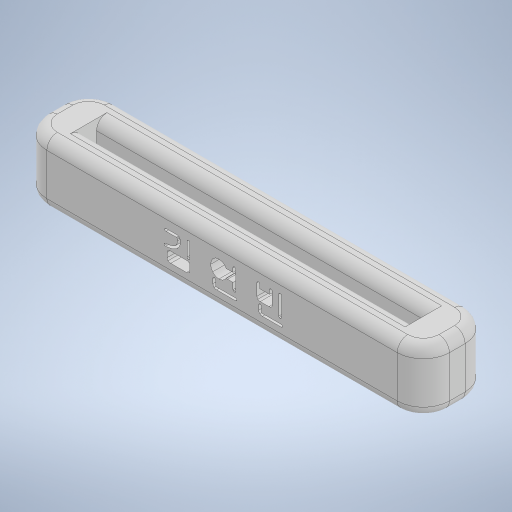
# Autodesk Inventor part: part2
Saved by Autodesk Inventor 2024 (Build 280153000, 153)
## iProperties
Created: 2023-11-09
Part Number: part2
Material: 일반
Document SubType Name: Modeling
Designer: SSAFY
Density: 1 g/cm^3
Appearance: 기본값
Author: SSAFY
Autodesk Inventor part; units mm, degrees
ref_plane "YZ Plane" through (0, 0, 0) normal (1, 0, 0) x (0, 1, 0)
ref_plane "XZ Plane" through (0, 0, 0) normal (0, 1, 0) x (-1, 0, 0)
ref_plane "XY Plane" through (0, 0, 0) normal (0, 0, 1) x (1, 0, 0)
sketch "스케치1" plane through (0, 0, 0) normal (0, 0, 1) x (1, 0, 0)
  point P0 (0, 0)
sketch "스케치2" plane through (0, 0, 0) normal (0, 1, 0) x (-1, 0, 0)
  line L0 (-38.5, 6.5) -> (38.5, 6.5)
  line L1 (38.5, 6.5) -> (38.5, -6.5)
  line L2 (38.5, -6.5) -> (-38.5, -6.5)
  line L3 (-38.5, -6.5) -> (-38.5, 6.5)
  line L4 (-38.5, 6.5) -> (38.5, -6.5) construction
  line L5 (38.5, 6.5) -> (-38.5, -6.5) construction
  line L6 (-32, 1.5) -> (32, 1.5)
  line L7 (32, 1.5) -> (32, -1.5)
  line L8 (32, -1.5) -> (-32, -1.5)
  line L9 (-32, -1.5) -> (-32, 1.5)
  line L10 (-32, 1.5) -> (32, -1.5) construction
  line L11 (32, 1.5) -> (-32, -1.5) construction
  point P0 (0, 0)
  dimension "d0" = 77
  dimension "d1" = 13
  dimension "d2" = 64
  dimension "d3" = 3
  constraints: 24 end point, 4 midpoint, 4 parallel, 2 horizontal, 2 perpendicular
  measures "d0" distance of L1.end L2.end
  measures "d1" distance of L2.end L0.start
  measures "d2" distance of L7.end L8.end
  measures "d3" distance of L8.end L6.start
extrude "돌출1" add sketch "스케치2" along normal mid plane 12
fillet "모깎기1" radius 5 4 edges at (38.5, 0, 6.5) (38.5, 0, -6.5) (-38.5, 0, 6.5) (-38.5, 0, -6.5)
fillet "모깎기2" radius 2 20 edges at (0, 6, 1.5) (0, -6, 1.5) (0, -6, -1.5) (0, 6, -1.5) (-37.0355, 6, -5.0355) (-38.5, 6, 0) (-37.0355, 6, 5.0355) (0, 6, 6.5) (37.0355, 6, 5.0355) (38.5, 6, 0) (37.0355, 6, -5.0355) (0, 6, -6.5) (37.0355, -6, -5.0355) (38.5, -6, 0) (37.0355, -6, 5.0355) (0, -6, 6.5) (-37.0355, -6, 5.0355) (-38.5, -6, 0) (-37.0355, -6, -5.0355) (0, -6, -6.5)
sketch "스케치3" plane through (-33.5, -4, 6.5) normal (0, 0, 1) x (1, 0, 0)
  line L0 (17.2421, 7.3141) -> (50.5083, 7.3141) construction
  line L1 (50.5083, 7.3141) -> (50.5083, 0.4358) construction
  line L2 (50.5083, 0.4358) -> (17.2421, 0.4358) construction
  line L3 (17.2421, 0.4358) -> (17.2421, 7.3141) construction
  line L4 (26.7014, 3.1578) -> (23.6098, 3.1578)
  spline S0 degree 2 poles (23.6098, 3.1578) (23.3343, 3.1578) (23.1722, 2.9997) knots 0 0 0 1 1 1
  spline S1 degree 2 poles (23.1722, 2.9997) (23.0061, 2.8417) (23.0061, 2.6067) knots 0 0 0 1 1 1
  line L5 (23.0061, 2.6067) -> (23.0061, 1.7396)
  spline S2 degree 2 poles (23.0061, 1.7396) (23.0061, 1.4479) (23.1641, 1.2939) knots 0 0 0 1 1 1
  spline S3 degree 2 poles (23.1641, 1.2939) (23.3343, 1.1318) (23.6949, 1.1318) knots 0 0 0 1 1 1
  line L6 (23.6949, 1.1318) -> (26.7297, 1.1318)
  spline S4 degree 2 poles (26.7297, 1.1318) (27.0174, 1.1318) (27.2119, 1.3749) knots 0 0 0 1 1 1
  spline S5 degree 2 poles (27.2119, 1.3749) (27.3699, 1.4236) (27.3699, 1.7072) knots 0 0 0 1 1 1
  line L7 (27.3699, 1.7072) -> (27.3699, 2.631)
  spline S6 degree 2 poles (27.3699, 2.631) (27.3699, 2.8701) (27.2119, 2.9997) knots 0 0 0 1 1 1
  spline S7 degree 2 poles (27.2119, 2.9997) (27.0012, 3.1578) (26.7014, 3.1578) knots 0 0 0 1 1 1
  line L8 (26.8351, 2.5338) -> (26.8351, 1.7477)
  spline S8 degree 2 poles (26.8351, 1.7477) (26.8351, 1.6667) (26.8027, 1.6424) knots 0 0 0 1 1 1
  spline S9 degree 2 poles (26.8027, 1.6424) (26.7419, 1.6018) (26.6163, 1.6018) knots 0 0 0 1 1 1
  line L9 (26.6163, 1.6018) -> (23.7678, 1.6018)
  spline S10 degree 2 poles (23.7678, 1.6018) (23.6219, 1.6018) (23.5733, 1.6424) knots 0 0 0 1 1 1
  spline S11 degree 2 poles (23.5733, 1.6424) (23.5409, 1.6707) (23.5409, 1.7761) knots 0 0 0 1 1 1
  line L10 (23.5409, 1.7761) -> (23.5409, 2.5176)
  spline S12 degree 2 poles (23.5409, 2.5176) (23.5409, 2.6148) (23.5814, 2.6553) knots 0 0 0 1 1 1
  spline S13 degree 2 poles (23.5814, 2.6553) (23.6179, 2.6877) (23.7475, 2.6877) knots 0 0 0 1 1 1
  line L11 (23.7475, 2.6877) -> (26.6082, 2.6877)
  spline S14 degree 2 poles (26.6082, 2.6877) (26.7419, 2.6877) (26.8027, 2.6472) knots 0 0 0 1 1 1
  spline S15 degree 2 poles (26.8027, 2.6472) (26.8351, 2.6229) (26.8351, 2.5338) knots 0 0 0 1 1 1
  line L12 (24.8051, 6.46) -> (22.7913, 6.46)
  spline S16 degree 2 poles (22.7913, 6.46) (22.536, 6.46) (22.5441, 6.2291) knots 0 0 0 1 1 1
  spline S17 degree 2 poles (22.5441, 6.2291) (22.5441, 5.99) (22.7954, 5.99) knots 0 0 0 1 1 1
  line L13 (22.7954, 5.99) -> (24.7646, 5.99)
  spline S18 degree 2 poles (24.7646, 5.99) (24.878, 5.99) (24.9307, 5.9454) knots 0 0 0 1 1 1
  spline S19 degree 2 poles (24.9307, 5.9454) (24.9996, 5.8928) (24.9996, 5.7874) knots 0 0 0 1 1 1
  line L14 (24.9996, 5.7874) -> (24.9996, 5.4997)
  spline S20 degree 2 poles (24.9996, 5.4997) (24.9996, 4.7907) (24.489, 4.4098) knots 0 0 0 1 1 1
  spline S21 degree 2 poles (24.489, 4.4098) (23.8286, 4.0046) (22.7305, 3.96) knots 0 0 0 1 1 1
  spline S22 degree 2 poles (22.7305, 3.96) (22.5766, 3.96) (22.4996, 3.883) knots 0 0 0 1 1 1
  spline S23 degree 2 poles (22.4996, 3.883) (22.4347, 3.8142) (22.4347, 3.7169) knots 0 0 0 1 1 1
  spline S24 degree 2 poles (22.4347, 3.7169) (22.4347, 3.6156) (22.5198, 3.5508) knots 0 0 0 1 1 1
  spline S25 degree 2 poles (22.5198, 3.5508) (22.5968, 3.49) (22.7224, 3.49) knots 0 0 0 1 1 1
  spline S26 degree 2 poles (22.7224, 3.49) (24.0393, 3.5508) (24.7727, 4.0816) knots 0 0 0 1 1 1
  spline S27 degree 2 poles (24.7727, 4.0816) (25.5142, 4.6164) (25.5142, 5.4957) knots 0 0 0 1 1 1
  line L15 (25.5142, 5.4957) -> (25.5142, 5.8441)
  spline S28 degree 2 poles (25.5142, 5.8441) (25.5142, 6.1197) (25.2994, 6.298) knots 0 0 0 1 1 1
  spline S29 degree 2 poles (25.2994, 6.298) (25.109, 6.46) (24.8051, 6.46) knots 0 0 0 1 1 1
  line L16 (27.3699, 3.7493) -> (27.3699, 6.3749)
  spline S30 degree 2 poles (27.3699, 6.3749) (27.3699, 6.4924) (27.2767, 6.5573) knots 0 0 0 1 1 1
  spline S31 degree 2 poles (27.2767, 6.5573) (27.2078, 6.6181) (27.1025, 6.6181) knots 0 0 0 1 1 1
  spline S32 degree 2 poles (27.1025, 6.6181) (26.989, 6.6181) (26.9161, 6.5573) knots 0 0 0 1 1 1
  spline S33 degree 2 poles (26.9161, 6.5573) (26.8351, 6.4803) (26.8351, 6.3709) knots 0 0 0 1 1 1
  line L17 (26.8351, 6.3709) -> (26.8351, 3.7493)
  spline S34 degree 2 poles (26.8351, 3.7493) (26.8351, 3.6278) (26.9121, 3.5508) knots 0 0 0 1 1 1
  spline S35 degree 2 poles (26.9121, 3.5508) (26.985, 3.4779) (27.1025, 3.4779) knots 0 0 0 1 1 1
  spline S36 degree 2 poles (27.1025, 3.4779) (27.2119, 3.4779) (27.2929, 3.5589) knots 0 0 0 1 1 1
  spline S37 degree 2 poles (27.2929, 3.5589) (27.3699, 3.6278) (27.3699, 3.7493) knots 0 0 0 1 1 1
  spline S38 degree 2 poles (32.921, 6.4479) (32.1714, 6.4479) (31.7297, 5.9292) knots 0 0 0 1 1 1
  spline S39 degree 2 poles (31.7297, 5.9292) (31.3367, 5.4714) (31.3367, 4.8028) knots 0 0 0 1 1 1
  spline S40 degree 2 poles (31.3367, 4.8028) (31.3367, 4.1383) (31.7135, 3.7412) knots 0 0 0 1 1 1
  spline S41 degree 2 poles (31.7135, 3.7412) (32.1714, 3.1537) (32.921, 3.1537) knots 0 0 0 1 1 1
  spline S42 degree 2 poles (32.921, 3.1537) (33.6584, 3.1537) (34.092, 3.6723) knots 0 0 0 1 1 1
  spline S43 degree 2 poles (34.092, 3.6723) (34.485, 4.1343) (34.485, 4.8028) knots 0 0 0 1 1 1
  spline S44 degree 2 poles (34.485, 4.8028) (34.485, 5.4714) (34.092, 5.9292) knots 0 0 0 1 1 1
  spline S45 degree 2 poles (34.092, 5.9292) (33.6584, 6.4479) (32.921, 6.4479) knots 0 0 0 1 1 1
  spline S46 degree 2 poles (32.921, 5.9779) (33.4193, 5.9779) (33.6989, 5.6213) knots 0 0 0 1 1 1
  spline S47 degree 2 poles (33.6989, 5.6213) (33.9664, 5.289) (33.9664, 4.8028) knots 0 0 0 1 1 1
  spline S48 degree 2 poles (33.9664, 4.8028) (33.9664, 4.3125) (33.6949, 3.9762) knots 0 0 0 1 1 1
  spline S49 degree 2 poles (33.6949, 3.9762) (33.4193, 3.6237) (32.921, 3.6237) knots 0 0 0 1 1 1
  spline S50 degree 2 poles (32.921, 3.6237) (32.4104, 3.6237) (32.1268, 3.9884) knots 0 0 0 1 1 1
  spline S51 degree 2 poles (32.1268, 3.9884) (31.8715, 4.3085) (31.8715, 4.8028) knots 0 0 0 1 1 1
  spline S52 degree 2 poles (31.8715, 4.8028) (31.8715, 5.2931) (32.1268, 5.6172) knots 0 0 0 1 1 1
  spline S53 degree 2 poles (32.1268, 5.6172) (32.4145, 5.9779) (32.921, 5.9779) knots 0 0 0 1 1 1
  line L18 (36.13, 2.7404) -> (36.13, 6.3749)
  spline S54 degree 2 poles (36.13, 6.3749) (36.13, 6.4924) (36.0409, 6.5532) knots 0 0 0 1 1 1
  spline S55 degree 2 poles (36.0409, 6.5532) (35.968, 6.6181) (35.8626, 6.6181) knots 0 0 0 1 1 1
  spline S56 degree 2 poles (35.8626, 6.6181) (35.7492, 6.6181) (35.6762, 6.5573) knots 0 0 0 1 1 1
  spline S57 degree 2 poles (35.6762, 6.5573) (35.5952, 6.4843) (35.5952, 6.3709) knots 0 0 0 1 1 1
  line L19 (35.5952, 6.3709) -> (35.5952, 5.5929)
  line L20 (35.5952, 5.5929) -> (34.5417, 5.5929)
  spline S58 degree 2 poles (34.5417, 5.5929) (34.4121, 5.5929) (34.3391, 5.5281) knots 0 0 0 1 1 1
  spline S59 degree 2 poles (34.3391, 5.5281) (34.2743, 5.4552) (34.2743, 5.3539) knots 0 0 0 1 1 1
  spline S60 degree 2 poles (34.2743, 5.3539) (34.2824, 5.2647) (34.3513, 5.1958) knots 0 0 0 1 1 1
  spline S61 degree 2 poles (34.3513, 5.1958) (34.4445, 5.1229) (34.5741, 5.1229) knots 0 0 0 1 1 1
  line L21 (34.5741, 5.1229) -> (35.5952, 5.1229)
  line L22 (35.5952, 5.1229) -> (35.5952, 4.3936)
  line L23 (35.5952, 4.3936) -> (34.5539, 4.3936)
  spline S62 degree 2 poles (34.5539, 4.3936) (34.4323, 4.3936) (34.3472, 4.3287) knots 0 0 0 1 1 1
  spline S63 degree 2 poles (34.3472, 4.3287) (34.2824, 4.2639) (34.2824, 4.1667) knots 0 0 0 1 1 1
  spline S64 degree 2 poles (34.2824, 4.1667) (34.2824, 4.0654) (34.3594, 4.0005) knots 0 0 0 1 1 1
  spline S65 degree 2 poles (34.3594, 4.0005) (34.4364, 3.9317) (34.562, 3.9317) knots 0 0 0 1 1 1
  line L24 (34.562, 3.9317) -> (35.5952, 3.9317)
  line L25 (35.5952, 3.9317) -> (35.5952, 2.7404)
  spline S66 degree 2 poles (35.5952, 2.7404) (35.5952, 2.6108) (35.6722, 2.5338) knots 0 0 0 1 1 1
  spline S67 degree 2 poles (35.6722, 2.5338) (35.7451, 2.4608) (35.8626, 2.4608) knots 0 0 0 1 1 1
  spline S68 degree 2 poles (35.8626, 2.4608) (35.972, 2.4608) (36.0531, 2.5419) knots 0 0 0 1 1 1
  spline S69 degree 2 poles (36.0531, 2.5419) (36.13, 2.6108) (36.13, 2.7404) knots 0 0 0 1 1 1
  spline S70 degree 2 poles (32.2929, 2.6634) (32.2929, 2.7971) (32.2159, 2.866) knots 0 0 0 1 1 1
  spline S71 degree 2 poles (32.2159, 2.866) (32.1349, 2.9471) (32.0255, 2.9471) knots 0 0 0 1 1 1
  spline S72 degree 2 poles (32.0255, 2.9471) (31.908, 2.9471) (31.8351, 2.8741) knots 0 0 0 1 1 1
  spline S73 degree 2 poles (31.8351, 2.8741) (31.7581, 2.7971) (31.7581, 2.6634) knots 0 0 0 1 1 1
  line L26 (31.7581, 2.6634) -> (31.7581, 1.7882)
  spline S74 degree 2 poles (31.7581, 1.7882) (31.7581, 1.4641) (31.9728, 1.2858) knots 0 0 0 1 1 1
  spline S75 degree 2 poles (31.9728, 1.2858) (32.1552, 1.1318) (32.4793, 1.1318) knots 0 0 0 1 1 1
  line L27 (32.4793, 1.1318) -> (36.0936, 1.1318)
  spline S76 degree 2 poles (36.0936, 1.1318) (36.3286, 1.1318) (36.3286, 1.3709) knots 0 0 0 1 1 1
  spline S77 degree 2 poles (36.3286, 1.3709) (36.3286, 1.6018) (36.0936, 1.6018) knots 0 0 0 1 1 1
  line L28 (36.0936, 1.6018) -> (32.5482, 1.6018)
  spline S78 degree 2 poles (32.5482, 1.6018) (32.3821, 1.6018) (32.3456, 1.6343) knots 0 0 0 1 1 1
  spline S79 degree 2 poles (32.3456, 1.6343) (32.2929, 1.6869) (32.2929, 1.8409) knots 0 0 0 1 1 1
  line L29 (32.2929, 1.8409) -> (32.2929, 2.6634)
  line L30 (42.5887, 6.2048) -> (42.5887, 5.4471)
  line L31 (42.5887, 5.4471) -> (40.7046, 5.4471)
  line L32 (40.7046, 5.4471) -> (40.7046, 6.1723)
  spline S80 degree 2 poles (40.7046, 6.1723) (40.7046, 6.3061) (40.6276, 6.3749) knots 0 0 0 1 1 1
  spline S81 degree 2 poles (40.6276, 6.3749) (40.5466, 6.456) (40.4372, 6.456) knots 0 0 0 1 1 1
  spline S82 degree 2 poles (40.4372, 6.456) (40.3278, 6.456) (40.2629, 6.383) knots 0 0 0 1 1 1
  spline S83 degree 2 poles (40.2629, 6.383) (40.1779, 6.298) (40.1779, 6.1683) knots 0 0 0 1 1 1
  line L33 (40.1779, 6.1683) -> (40.1779, 3.9276)
  spline S84 degree 2 poles (40.1779, 3.9276) (40.1779, 3.6521) (40.344, 3.5062) knots 0 0 0 1 1 1
  spline S85 degree 2 poles (40.344, 3.5062) (40.5304, 3.3522) (40.8018, 3.3522) knots 0 0 0 1 1 1
  line L34 (40.8018, 3.3522) -> (42.455, 3.3522)
  spline S86 degree 2 poles (42.455, 3.3522) (42.7386, 3.3522) (42.9129, 3.5103) knots 0 0 0 1 1 1
  spline S87 degree 2 poles (42.9129, 3.5103) (43.1033, 3.6723) (43.1033, 3.9276) knots 0 0 0 1 1 1
  line L35 (43.1033, 3.9276) -> (43.1033, 6.2007)
  spline S88 degree 2 poles (43.1033, 6.2007) (43.1033, 6.456) (42.844, 6.456) knots 0 0 0 1 1 1
  spline S89 degree 2 poles (42.844, 6.456) (42.5887, 6.456) (42.5887, 6.2048) knots 0 0 0 1 1 1
  spline S90 degree 2 poles (41.0531, 2.6634) (41.0531, 2.7971) (40.9761, 2.866) knots 0 0 0 1 1 1
  spline S91 degree 2 poles (40.9761, 2.866) (40.895, 2.9471) (40.7856, 2.9471) knots 0 0 0 1 1 1
  spline S92 degree 2 poles (40.7856, 2.9471) (40.6681, 2.9471) (40.5952, 2.8741) knots 0 0 0 1 1 1
  spline S93 degree 2 poles (40.5952, 2.8741) (40.5182, 2.7971) (40.5182, 2.6634) knots 0 0 0 1 1 1
  line L36 (40.5182, 2.6634) -> (40.5182, 1.7882)
  spline S94 degree 2 poles (40.5182, 1.7882) (40.5182, 1.4641) (40.733, 1.2858) knots 0 0 0 1 1 1
  spline S95 degree 2 poles (40.733, 1.2858) (40.9153, 1.1318) (41.2394, 1.1318) knots 0 0 0 1 1 1
  line L37 (41.2394, 1.1318) -> (44.8537, 1.1318)
  spline S96 degree 2 poles (44.8537, 1.1318) (45.0887, 1.1318) (45.0887, 1.3709) knots 0 0 0 1 1 1
  spline S97 degree 2 poles (45.0887, 1.3709) (45.0887, 1.6018) (44.8537, 1.6018) knots 0 0 0 1 1 1
  line L38 (44.8537, 1.6018) -> (41.3083, 1.6018)
  spline S98 degree 2 poles (41.3083, 1.6018) (41.1422, 1.6018) (41.1057, 1.6343) knots 0 0 0 1 1 1
  spline S99 degree 2 poles (41.1057, 1.6343) (41.0531, 1.6869) (41.0531, 1.8409) knots 0 0 0 1 1 1
  line L39 (41.0531, 1.8409) -> (41.0531, 2.6634)
  line L40 (44.8902, 2.7404) -> (44.8902, 6.3749)
  spline S100 degree 2 poles (44.8902, 6.3749) (44.8902, 6.4924) (44.801, 6.5532) knots 0 0 0 1 1 1
  spline S101 degree 2 poles (44.801, 6.5532) (44.7281, 6.6181) (44.6228, 6.6181) knots 0 0 0 1 1 1
  spline S102 degree 2 poles (44.6228, 6.6181) (44.5093, 6.6181) (44.4364, 6.5573) knots 0 0 0 1 1 1
  spline S103 degree 2 poles (44.4364, 6.5573) (44.3553, 6.4803) (44.3553, 6.3709) knots 0 0 0 1 1 1
  line L41 (44.3553, 6.3709) -> (44.3553, 2.7404)
  spline S104 degree 2 poles (44.3553, 2.7404) (44.3553, 2.6108) (44.4323, 2.5338) knots 0 0 0 1 1 1
  spline S105 degree 2 poles (44.4323, 2.5338) (44.5052, 2.4608) (44.6228, 2.4608) knots 0 0 0 1 1 1
  spline S106 degree 2 poles (44.6228, 2.4608) (44.7322, 2.4608) (44.8132, 2.5419) knots 0 0 0 1 1 1
  spline S107 degree 2 poles (44.8132, 2.5419) (44.8902, 2.6108) (44.8902, 2.7404) knots 0 0 0 1 1 1
  line L42 (42.5887, 4.977) -> (42.5887, 4.0087)
  spline S108 degree 2 poles (42.5887, 4.0087) (42.5887, 3.9074) (42.5279, 3.8668) knots 0 0 0 1 1 1
  spline S109 degree 2 poles (42.5279, 3.8668) (42.4753, 3.8223) (42.3416, 3.8223) knots 0 0 0 1 1 1
  line L43 (42.3416, 3.8223) -> (40.9072, 3.8223)
  spline S110 degree 2 poles (40.9072, 3.8223) (40.7816, 3.8223) (40.7492, 3.8547) knots 0 0 0 1 1 1
  spline S111 degree 2 poles (40.7492, 3.8547) (40.7046, 3.8911) (40.7046, 4.0087) knots 0 0 0 1 1 1
  line L44 (40.7046, 4.0087) -> (40.7046, 4.977)
  line L45 (40.7046, 4.977) -> (42.5887, 4.977)
  point P0 (33.5, 4)
  constraints: 2 other
emboss "엠보싱1" sketch "스케치3" operation cut depth 5 direction (0, 0, -1) contours S7 S6 L7 S5 S4 L6 S3 S2 L5 S1 S0 L4 | S29 S28 L15 S27 S26 S25 S24 S23 S22 S21 S20 L14 S19 S18 L13 S17 S16 L12 | S37 S36 S35 S34 L17 S33 S32 S31 S30 L16 | S45 S44 S58 S59 S60 S61 S43 S62 S63 S64 S42 S41 S40 S39 S38 | S58 L20 L19 S57 S56 S55 S54 L18 S69 S68 S67 S66 L25 L24 S65 S64 S43 S62 L23 L22 L21 S61 S44 | S44 S61 S60 S59 S58 | S43 S64 S63 S62 | L29 S79 S78 L28 S77 S76 L27 S75 S74 L26 S73 S72 S71 S70 | S89 S88 L35 S87 S86 L34 S85 S84 L33 S83 S82 S81 S80 L32 L31 L30 | L39 S99 S98 L38 S97 S96 L37 S95 S94 L36 S93 S92 S91 S90 | S107 S106 S105 S104 L41 S103 S102 S101 S100 L40
sketch "스케치4" plane through (-33.5, -4, 6.5) normal (0, 0, 1) x (1, 0, 0)
  spline S0 degree 5 poles (23.5733, 1.6424) (23.593, 1.6259) (23.6227, 1.6137) (23.662, 1.6057) (23.7106, 1.6018) (23.7678, 1.6018) knots 0 0 0 0 0 0 1 1 1 1 1 1 projected
  line L0 (23.7678, 1.6018) -> (26.6163, 1.6018) projected
  spline S1 degree 5 poles (26.6163, 1.6018) (26.6659, 1.6018) (26.7096, 1.6058) (26.7471, 1.6138) (26.7781, 1.626) (26.8027, 1.6424) knots 0 0 0 0 0 0 1 1 1 1 1 1 projected
  spline S2 degree 5 poles (26.8027, 1.6424) (26.8157, 1.6521) (26.8254, 1.6676) (26.8319, 1.6887) (26.8351, 1.7155) (26.8351, 1.7477) knots 0 0 0 0 0 0 1 1 1 1 1 1 projected
  line L1 (26.8351, 1.7477) -> (26.8351, 2.5338) projected
  spline S3 degree 5 poles (26.8351, 2.5338) (26.8351, 2.5691) (26.8319, 2.5983) (26.8254, 2.6212) (26.8157, 2.6375) (26.8027, 2.6472) knots 0 0 0 0 0 0 1 1 1 1 1 1 projected
  spline S4 degree 5 poles (26.8027, 2.6472) (26.7781, 2.6636) (26.7462, 2.6758) (26.707, 2.6838) (26.6609, 2.6877) (26.6082, 2.6877) knots 0 0 0 0 0 0 1 1 1 1 1 1 projected
  line L2 (26.6082, 2.6877) -> (23.7475, 2.6877) projected
  spline S5 degree 5 poles (23.7475, 2.6877) (23.6966, 2.6877) (23.654, 2.6846) (23.6204, 2.6782) (23.5962, 2.6684) (23.5814, 2.6553) knots 0 0 0 0 0 0 1 1 1 1 1 1 projected
  spline S6 degree 5 poles (23.5814, 2.6553) (23.5651, 2.639) (23.553, 2.6171) (23.5449, 2.5894) (23.5409, 2.5562) (23.5409, 2.5176) knots 0 0 0 0 0 0 1 1 1 1 1 1 projected
  line L3 (23.5409, 2.5176) -> (23.5409, 1.7761) projected
  spline S7 degree 5 poles (23.5409, 1.7761) (23.5409, 1.7344) (23.5441, 1.6999) (23.5505, 1.673) (23.5603, 1.6538) (23.5733, 1.6424) knots 0 0 0 0 0 0 1 1 1 1 1 1 projected
  line L4 (34.5539, 4.3936) -> (35.5952, 4.3936) projected
  line L5 (35.5952, 4.3936) -> (35.5952, 5.1229) projected
  line L6 (35.5952, 5.1229) -> (34.5741, 5.1229) projected
  spline S8 degree 4 poles (34.5741, 5.1229) (34.543, 5.1229) (34.5133, 5.1257) (34.4849, 5.1313) (34.4578, 5.1398) knots 0 0 0 0 0 1 1 1 1 1 projected
  spline S9 degree 6 poles (34.4578, 5.1398) (34.4671, 5.0849) (34.4744, 5.0294) (34.4797, 4.9734) (34.4833, 4.9169) (34.485, 4.86) (34.485, 4.8028) knots 0 0 0 0 0 0 0 1 1 1 1 1 1 1 projected
  spline S10 degree 6 poles (34.485, 4.8028) (34.485, 4.7301) (34.4822, 4.658) (34.4765, 4.5864) (34.4677, 4.5157) (34.4558, 4.4459) (34.4407, 4.3771) knots 0 0 0 0 0 0 0 1 1 1 1 1 1 1 projected
  spline S11 degree 4 poles (34.4407, 4.3771) (34.4667, 4.3854) (34.4943, 4.3909) (34.5234, 4.3936) (34.5539, 4.3936) knots 0 0 0 0 0 1 1 1 1 1 projected
  spline S12 degree 5 poles (32.921, 3.6237) (32.9619, 3.6237) (33.0025, 3.6252) (33.0424, 3.6283) (33.0818, 3.6329) (33.196, 3.6516) (33.2688, 3.6704) (33.3385, 3.6959) (33.4045, 3.7282) (33.5182, 3.8001) (33.5673, 3.8376) (33.6131, 3.8797) (33.6557, 3.9261) (33.6949, 3.9762) knots 0 0 0 0 0 0 0.217529 0.217529 0.217529 0.217529 0.642132 0.642132 0.642132 0.642132 1 1 1 1 1 1 projected
  spline S13 degree 6 poles (33.6949, 3.9762) (33.7152, 4.0015) (33.7348, 4.0273) (33.7534, 4.0537) (33.7711, 4.0806) (33.7879, 4.1081) (33.8591, 4.234) (33.9032, 4.3383) (33.9356, 4.4483) (33.9564, 4.563) (33.9664, 4.6815) (33.9664, 4.8028) knots 0 0 0 0 0 0 0 0.222523 0.222523 0.222523 0.222523 0.222523 1 1 1 1 1 1 1 projected
  spline S14 degree 6 poles (33.9664, 4.8028) (33.9664, 4.9249) (33.9562, 5.0441) (33.9351, 5.1594) (33.9023, 5.2697) (33.8574, 5.3742) (33.7861, 5.4981) (33.7703, 5.5238) (33.7536, 5.5489) (33.7362, 5.5735) (33.7179, 5.5977) (33.6989, 5.6213) knots 0 0 0 0 0 0 0 0.789429 0.789429 0.789429 0.789429 0.789429 1 1 1 1 1 1 1 projected
  spline S15 degree 5 poles (33.6989, 5.6213) (33.6577, 5.6739) (33.6128, 5.7224) (33.5645, 5.7663) (33.5127, 5.8052) (33.3962, 5.8768) (33.3308, 5.9082) (33.2618, 5.9329) (33.1897, 5.9511) (33.0775, 5.9691) (33.0391, 5.9735) (33.0002, 5.9764) (32.9608, 5.9779) (32.921, 5.9779) knots 0 0 0 0 0 0 0.372291 0.372291 0.372291 0.372291 0.789043 0.789043 0.789043 0.789043 1 1 1 1 1 1 projected
  spline S16 degree 5 poles (32.921, 5.9779) (32.8805, 5.9779) (32.8404, 5.9764) (32.8008, 5.9735) (32.7618, 5.969) (32.6479, 5.9508) (32.5749, 5.9326) (32.5048, 5.9078) (32.4382, 5.8763) (32.319, 5.8041) (32.2657, 5.7646) (32.2158, 5.72) (32.1695, 5.6708) (32.1268, 5.6172) knots 0 0 0 0 0 0 0.210952 0.210952 0.210952 0.210952 0.625739 0.625739 0.625739 0.625739 1 1 1 1 1 1 projected
  spline S17 degree 6 poles (32.1268, 5.6172) (32.1164, 5.6041) (32.1063, 5.5907) (32.0964, 5.5772) (32.0868, 5.5635) (32.0774, 5.5497) (32.0009, 5.4321) (31.9473, 5.3194) (31.9083, 5.1988) (31.8834, 5.0715) (31.8715, 4.9391) (31.8715, 4.8028) knots 0 0 0 0 0 0 0 0.119158 0.119158 0.119158 0.119158 0.119158 1 1 1 1 1 1 1 projected
  spline S18 degree 5 poles (31.8715, 4.8028) (31.8715, 4.7164) (31.8764, 4.6317) (31.8865, 4.5491) (31.9022, 4.4689) (31.9441, 4.3179) (31.9698, 4.2468) (32.0009, 4.1787) (32.0375, 4.114) (32.0883, 4.0396) (32.0975, 4.0265) (32.107, 4.0136) (32.1168, 4.0009) (32.1268, 3.9884) knots 0 0 0 0 0 0 0.463178 0.463178 0.463178 0.463178 0.90457 0.90457 0.90457 0.90457 1 1 1 1 1 1 projected
  spline S19 degree 5 poles (32.1268, 3.9884) (32.1682, 3.9351) (32.2132, 3.886) (32.2618, 3.8415) (32.3139, 3.8019) (32.4321, 3.7284) (32.4992, 3.6959) (32.5699, 3.6704) (32.6438, 3.6516) (32.7592, 3.6329) (32.7988, 3.6282) (32.8391, 3.6252) (32.8798, 3.6237) (32.921, 3.6237) knots 0 0 0 0 0 0 0.368015 0.368015 0.368015 0.368015 0.786619 0.786619 0.786619 0.786619 1 1 1 1 1 1 projected
  line L7 (40.9072, 3.8223) -> (42.3416, 3.8223) projected
  spline S20 degree 5 poles (42.3416, 3.8223) (42.3942, 3.8223) (42.4396, 3.8266) (42.4772, 3.8354) (42.5067, 3.8488) (42.5279, 3.8668) knots 0 0 0 0 0 0 1 1 1 1 1 1 projected
  spline S21 degree 5 poles (42.5279, 3.8668) (42.532, 3.8695) (42.5358, 3.8724) (42.5395, 3.8754) (42.5431, 3.8786) (42.5634, 3.8989) (42.5761, 3.9201) (42.5845, 3.9455) (42.5887, 3.9751) (42.5887, 4.0087) knots 0 0 0 0 0 0 0.165558 0.165558 0.165558 0.165558 1 1 1 1 1 1 projected
  line L8 (42.5887, 4.0087) -> (42.5887, 4.977) projected
  line L9 (42.5887, 4.977) -> (40.7046, 4.977) projected
  line L10 (40.7046, 4.977) -> (40.7046, 4.0087) projected
  spline S22 degree 5 poles (40.7046, 4.0087) (40.7046, 3.9622) (40.7089, 3.9233) (40.7178, 3.8923) (40.7312, 3.8694) (40.7492, 3.8547) knots 0 0 0 0 0 0 1 1 1 1 1 1 projected
  spline S23 degree 5 poles (40.7492, 3.8547) (40.7623, 3.8416) (40.7849, 3.8318) (40.8168, 3.8254) (40.8578, 3.8223) (40.9072, 3.8223) knots 0 0 0 0 0 0 1 1 1 1 1 1 projected
  point P0 (33.5, 4)
  constraints: 24 other
extrude "돌출2" cut sketch "스케치4" against normal blind 6
